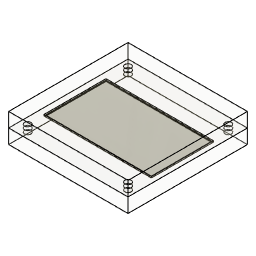
AcrylicBusinessCardHolders v7 (Autodesk Fusion 360 design; units mm, degrees)
Autodesk Fusion 360 part; units mm, degrees
sketch "Sketch1" plane through (0, 0, 0) normal (0, 0, 1) x (1, 0, 0)
  line L0 (0, 0) -> (100, 0)
  line L1 (100, 0) -> (100, 100)
  line L2 (100, 100) -> (0, 100)
  line L3 (0, 100) -> (0, 0)
  dimension "d1" = 100
  dimension "d2" = 100
  constraint horizontal L0
  constraint vertical L1
  constraint horizontal L2
  constraint vertical L3
  constraint coincident L0.start L3.end
  measures "d1" distance of L0.start L0.end
  measures "d2" distance of L0.start L2.end
extrude "Extrude1" add sketch "Sketch1" along normal blind 12 makes body 1
sketch "Sketch2" plane through (0, 0, 12) normal (0, 0, 1) x (-1, 0, 0)
  line L0 (0, -100) -> (0, 0)
  line L1 (0, 0) -> (-100, 0)
  line L2 (-100, 0) -> (-100, -100)
  line L3 (-100, -100) -> (0, -100)
  line L4 (-8, -8) -> (-92, -8) construction
  line L5 (-92, -8) -> (-92, -92) construction
  line L6 (-92, -92) -> (-8, -92) construction
  line L7 (-8, -92) -> (-8, -8) construction
  circle A0 centre (-8, -92) radius 2.675
  circle A1 centre (-92, -92) radius 2.675
  circle A2 centre (-8, -8) radius 2.675
  circle A3 centre (-92, -8) radius 2.675
  line L8 (-5, -76.5746) -> (-95, -76.5746)
  line L9 (-95, -76.5746) -> (-95, -24.5746)
  line L10 (-95, -24.5746) -> (-5, -24.5746)
  line L11 (-5, -24.5746) -> (-5, -76.5746)
  dimension "d5" = -8
  dimension "d6" = 5.35
  dimension "d7" = 5.35
  dimension "d8" = 5.35
  dimension "d9" = 5.35
  dimension "d10" = 52
  dimension "d11" = 90
  dimension "d12" = 5
  constraint coincident L6.end L7.start
  constraint coincident L5.end L6.start
  constraint coincident L4.start L7.end
  constraint coincident L4.end L5.start
  constraint horizontal L8
  constraint vertical L9
  constraint horizontal L10
  constraint vertical L11
  measures "d6" diameter of A0
  measures "d7" diameter of A1
  measures "d8" diameter of A2
  measures "d9" diameter of A3
  measures "d10" distance of L8 L10
  measures "d11" distance of L8.start L8.end
  measures "d12" distance of L0 L11
extrude "Extrude2" cut sketch "Sketch2" against normal blind 3 contours A0 | A1 | A2 | A3 bodies 1
extrude "Extrude3" cut sketch "Sketch2" against normal blind 1 contours L8 L9 L10 L11 bodies 1
sketch "Sketch3" plane through (0, 0, 11) normal (0, 0, 1) x (-1, 0, 0)
  line L0 (-5, -24.5746) -> (-95, -24.5746)
  line L1 (-95, -24.5746) -> (-95, -76.5746)
  line L2 (-95, -76.5746) -> (-5, -76.5746)
  line L3 (-5, -76.5746) -> (-5, -24.5746)
  line L4 (-6, -75.5746) -> (-94, -75.5746)
  line L5 (-94, -75.5746) -> (-94, -25.5746)
  line L6 (-94, -25.5746) -> (-6, -25.5746)
  line L7 (-6, -25.5746) -> (-6, -75.5746)
  dimension "d17" = 88
  dimension "d18" = 50
  dimension "d19" = 1
  dimension "d20" = 1
  constraint horizontal L4
  constraint vertical L5
  constraint horizontal L6
  constraint vertical L7
  measures "d17" distance of L4.start L4.end
  measures "d18" distance of L4.start L6.end
  measures "d19" distance of L2 L4
  measures "d20" distance of L3 L7
extrude "Extrude4" add sketch "Sketch3" along normal blind 0.3 separate body contours L4 L5 L6 L7 makes body 2
sketch "Sketch4" plane through (0, 0, 12) normal (0, 0, 1) x (-1, 0, 0)
  line L0 (-95, -76.5746) -> (-95, -24.5746)
  line L1 (-95, -24.5746) -> (-5, -24.5746)
  line L2 (-5, -24.5746) -> (-5, -76.5746)
  line L3 (-5, -76.5746) -> (-95, -76.5746)
  circle A0 centre (-92, -92) radius 2.675
  circle A1 centre (-92, -8) radius 2.675
  circle A2 centre (-8, -92) radius 2.675
  circle A3 centre (-8, -8) radius 2.675
  line L4 (0, -100) -> (0, 0)
  line L5 (0, 0) -> (-100, 0)
  line L6 (-100, 0) -> (-100, -100)
  line L7 (-100, -100) -> (0, -100)
  line L8 (0, -100) -> (-100, -100)
  line L9 (-100, -100) -> (-100, 0)
  line L10 (-100, 0) -> (0, 0)
  line L11 (0, 0) -> (0, -100)
  circle A4 centre (-8, -92) radius 2.5
  circle A5 centre (-92, -92) radius 2.5
  circle A6 centre (-92, -8) radius 2.5
  circle A7 centre (-8, -8) radius 2.5
  constraint horizontal L8
  constraint vertical L9
  constraint horizontal L10
  constraint vertical L11
  constraint coincident L5.end L6.start
  constraint coincident L4.start L7.end
  constraint concentric A2 A4
  constraint concentric A0 A5
  constraint concentric A1 A6
  constraint concentric A3 A7
extrude "Extrude5" add sketch "Sketch4" along normal blind 12 separate body contours L0 L1 L2 L3 | A0 | A1 | A2 | A3 | L4 L5 L6 L7 L8 L9 L10 L11 | A4 | A5 | A6 | A7 makes body 3
extrude "Extrude6" cut sketch "Sketch4" along normal blind 2.75 contours A0 | A1 | A2 | A3 | A4 | A5 | A6 | A7 bodies 3
